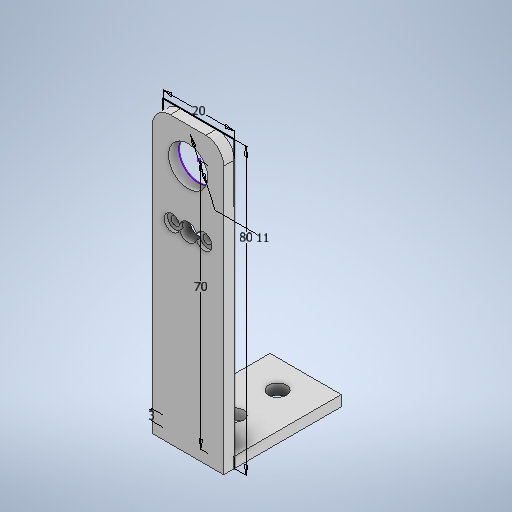
# Autodesk Inventor part: roll stand 1
Saved by Autodesk Inventor 2025.1 (Build 291241020, 241B)
## iProperties
Created: 2025-01-25
Part Number: roll stand 1
Material: Generic
Document SubType Name: Modeling
Designer: User
Density: 1 g/cm^3
Appearance: Default
Author: User
Autodesk Inventor part; units mm, degrees
ref_plane "YZ Plane" through (0, 0, 0) normal (1, 0, 0) x (0, 1, 0)
ref_plane "XZ Plane" through (0, 0, 0) normal (0, 1, 0) x (-1, 0, 0)
ref_plane "XY Plane" through (0, 0, 0) normal (0, 0, 1) x (1, 0, 0)
sketch "Sketch1" plane through (0, 0, 0) normal (0, 0, 1) x (1, 0, 0)
  line L0 (0, 0) -> (20, 0)
  line L1 (20, 0) -> (20, 80)
  line L2 (20, 80) -> (0, 80)
  line L3 (0, 80) -> (0, 0)
  circle A0 centre (10, 70) radius 5.5
  line L4 (20, 0) -> (0, 0)
  line L5 (0, 0) -> (0, 3)
  line L6 (0, 3) -> (20, 3)
  line L7 (20, 3) -> (20, 0)
  point P0 (10, 0)
  dimension "d0" = 20
  dimension "d1" = 80
  dimension "d2" = 11
  dimension "d3" = 70
  dimension "d7" = 3
  constraints: 16 end point, 4 parallel, 2 horizontal, 2 perpendicular, 1 centre point, 1 midpoint, 1 point on line
  measures "d0" distance of L2.end L1.end
  measures "d1" distance of L0.end L1.end
  measures "d2" diameter of A0
  measures "d3" distance of point (10, 0) A0.centre
  measures "d7" distance between parallel lines of L0 L6
extrude "Extrusion1" add sketch "Sketch1" along normal blind 3
fillet "Fillet1" radius 5 2 edges at (20, 80, 1.5) (0, 80, 1.5)
extrude "Extrusion2" add sketch "Sketch1" against normal blind 30 contours L3 L6 L1 L0
sketch "Sketch2" plane through (0, 3, 0) normal (0, 1, 0) x (1, 0, 0)
  circle A0 centre (10, 22.1006) radius 2.5
  circle A1 centre (10, 10.048) radius 2.5
  point P0 (0, 0)
  dimension "d10" = 5
  dimension "d11" = 5
  constraints: 2 centre point
  measures "d10" diameter of A0
  measures "d11" diameter of A1
extrude "Extrusion3" cut sketch "Sketch2" against normal through all
extrude "Extrusion4" cut sketch "Sketch1" along normal blind 10 contours A0
extrude "Extrusion5" cut sketch "Sketch1" along normal blind 10 contours A0
sketch "Sketch3" plane through (0, 0, 3) normal (0, 0, 1) x (1, 0, 0)
  circle A0 centre (10, 53.969) radius 2.5
  circle A1 centre (10, 70) radius 5.5 projected
  circle A2 centre (14.5, 53.969) radius 2.25
  circle A3 centre (5.5, 53.969) radius 2.25
  point P0 (0, 0)
  point P1 (7.6181, 54.7282)
  point P2 (7.6181, 53.2098)
  point P3 (12.3819, 53.2098)
  point P4 (12.3819, 54.7282)
  dimension "d18" = 5
  dimension "d19" = 16.031
  dimension "d20" = 4.5
  dimension "d21" = 4.5
  dimension "d22" = 4.5
  dimension "d23" = 4.5
  constraints: 3 centre point
  measures "d18" diameter of A0
  measures "d19" distance of A0.centre A1.centre
  measures "d20" diameter of A2
  measures "d21" diameter of A3
  measures "d22" distance of A0.centre A3.centre
  measures "d23" distance of A2.centre A0.centre
extrude "Extrusion6" cut sketch "Sketch3" against normal blind 1 contours A0 A2 | A0 A2 | A2 A0 A3 | A3 A0 | A0 A3
extrude "Extrusion7" cut sketch "Sketch3" against normal through all contours A0 A2 | A2 A0 A3 | A3 A0 picked at (12.3432, 53.969) picked at (7.5921, 53.969)
sketch "Sketch4" plane through (0, 0, 2) normal (0, 0, 1) x (1, 0, 0)
  arc A0 (7.6181, 54.7282) -> (7.6181, 53.2098) centre (5.5, 53.969) ccw projected
  circle A1 centre (5.5, 53.969) radius 1.25
  arc A2 (12.3819, 53.2098) -> (12.3819, 54.7282) centre (14.5, 53.969) ccw projected
  circle A3 centre (14.5, 53.969) radius 1.25
  point P0 (0, 0)
  dimension "d28" = 2.5
  dimension "d29" = 2.5
  constraints: 2 centre point, 2 coincident
  measures "d28" diameter of A1
  measures "d29" diameter of A3
extrude "Extrusion8" cut sketch "Sketch4" against normal through all
body "Solid1"
